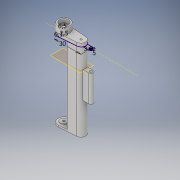
# Autodesk Inventor part: Servo-Arm-Lip
Saved by Autodesk Inventor 2018.3 (Build 223284000, 284)
## iProperties
Created: 2018-02-17
Part Number: Servo-Arm-Lip
Material: Generisch
Document SubType Name: Modeling
Designer: JochenAlt
Density: 1 g/cm^3
Appearance: Vorgabe
Author: JochenAlt
Autodesk Inventor part; units mm, degrees
ref_plane "YZ Plane" through (0, 0, 0) normal (1, 0, 0) x (0, 1, 0)
ref_plane "XZ Plane" through (0, 0, 0) normal (0, 1, 0) x (-1, 0, 0)
sketch "Skizze1" plane through (0, 0, 0) normal (0, 0, 1) x (1, 0, 0)
  line L0 (0, 5.6) -> (0, -5.6) construction
  line L1 (-9.12, 0) -> (26.72, 0) construction
  circle A0 centre (0, 0) radius 2
  circle A1 centre (9.5, 0) radius 1
  circle A2 centre (16, 0) radius 1
  circle A3 centre (19, 0) radius 1
  arc A4 (19.1916, -2.5929) -> (19.1916, 2.5929) centre (19, 0) ccw
  arc A5 (0.2947, 3.9891) -> (0.2947, -3.9891) centre (0, 0) ccw
  line L2 (0.2947, 3.9891) -> (19.1916, 2.5929)
  line L3 (0.2947, -3.9891) -> (19.1916, -2.5929)
  circle A6 centre (12.8, 0) radius 1
  circle A7 centre (0, 0) radius 4
  point P0 (0.5263, 3.9652)
  point P1 (0.6579, -1.8887)
  point P2 (0.6579, 1.8887)
  dimension "d0" = 9.5
  dimension "d1" = 16
  dimension "d2" = 19
  dimension "d3" = 5.2
  dimension "d4" = 2
  dimension "d5" = 4
  dimension "d6" = 8
  dimension "d17" = 12.8
  constraints: 7 centre point, 7 point on circle, 4 coincident, 4 end point, 4 point on line, 4 tangent, 3 equal radius, 3 other
  measures "d0" distance of A1.centre point (0, 0)
  measures "d1" distance of point (0, 0) A2.centre
  measures "d2" distance of A3.centre point (0, 0)
  measures "d3" diameter of A4
  measures "d4" diameter of A3
  measures "d5" diameter of A0
  measures "d6" diameter of A5
  measures "d17" distance of A6.centre point (0, 0)
extrude "Extrusion1" add sketch "Skizze1" along normal blind 1.8
extrude "Extrusion2" add sketch "Skizze1" against normal blind 2.7 contours A5 A7
sketch "Skizze6" plane through (0, 0, 0) normal (0, 0, 1) x (1, 0, 0)
  line L0 (0.2947, 3.9891) -> (19.1916, 2.5929) construction
  arc A0 (19.1916, -2.5929) -> (19.1916, 2.5929) centre (19, 0) ccw construction
  line L1 (19.1916, -2.5929) -> (0.2947, -3.9891) construction
  arc A1 (0.2947, -3.9891) -> (0.2947, 3.9891) centre (0, 0) ccw construction
  circle A2 centre (12.8, 0) radius 1 construction
  circle A3 centre (19, 0) radius 1 construction
  circle A4 centre (16, 0) radius 1 construction
  circle A5 centre (9.5, 0) radius 1 construction
  arc A6 (19.1989, -2.6927) -> (19.1989, 2.6927) centre (19, 0) ccw
  line L2 (19.1989, 2.6927) -> (0.3021, 4.0889)
  line L3 (19.3758, 5.0861) -> (0.4789, 6.4823)
  line L4 (0.4789, -6.4823) -> (19.3758, -5.0861)
  circle A7 centre (9.5, 0) radius 1 construction
  circle A8 centre (19, 0) radius 1
  line L5 (-21.489, 0) -> (83.4343, 0) construction
  arc A9 (0.4789, 6.4823) -> (0.4789, -6.4823) centre (0, 0) ccw
  arc A10 (0.3021, 4.0889) -> (0.3021, -4.0889) centre (0, 0) ccw
  line L6 (0.3021, -4.0889) -> (19.1989, -2.6927)
  circle A11 centre (0, 0) radius 2 construction
  circle A12 centre (0, 0) radius 4.1
  circle A13 centre (0, 0) radius 1.25
  arc A14 (19.3758, -5.0861) -> (19.3758, 5.0861) centre (19, 0) ccw
  line L7 (30, -2.5) -> (23.4452, -2.5)
  arc A15 (30, -2.5) -> (30, 2.5) centre (30, 0) ccw
  line L8 (23.4452, 2.5) -> (30, 2.5)
  circle A16 centre (30, 0) radius 1.5
  dimension "d106" = 2.5
  dimension "d116" = 0.1
  dimension "d198" = 6.5
  dimension "d203" = 5
  dimension "d204" = 30
  dimension "d205" = 3
  constraints: 12 end point, 12 point on circle, 11 centre point, 10 tangent, 8 coincident, 4 concentric, 3 parallel, 1 horizontal, 1 point on line, 1 other
  measures "d106" diameter of A13
  measures "d116" distance between parallel lines of L6 L1
  measures "d198" radius of A9
  measures "d203" diameter of A15
  measures "d204" distance of point (0, 0) A15.centre
  measures "d205" diameter of A16
extrude "Extrusion11" add sketch "Skizze6" along normal blind 2 separate body contours A14 L4 A9 L3
extrude "Extrusion12" add sketch "Skizze6" along normal blind 1.5 from surface at 2 contours L6 A12 L2 A6 | A10 A12 | A14 L4 A9 L3 | A13 bodies 2
extrude "Extrusion16" cut sketch "Skizze6" along normal up to next contours A13 bodies 2
ref_plane "Arbeitsebene8" through (0, 0, -6.75) normal (0, 0, 1) x (1, 0, 0)
sketch "Skizze18" plane through (0, 0, 3.5) normal (0, 0, 1) x (1, 0, 0)
  circle A0 centre (0, 0) radius 5
  circle A1 centre (0, 0) radius 6.5
  circle A2 centre (0, 0) radius 4
  dimension "d183" = 10
  dimension "d192" = 8
  dimension "d197" = 1.5
  constraints: 3 centre point, 3 coincident
  measures "d183" diameter of A0
  measures "d192" diameter of A2
  measures "d197" radial gap between concentric circles of A1 A0
extrude "Extrusion29" add sketch "Skizze18" along normal blind 3 contours A0 | A1 bodies 2
extrude "Extrusion28" add sketch "Skizze18" along normal blind 4 from surface at 3 contours A1 bodies 2
extrude "Extrusion30" add sketch "Skizze6" along normal up to surface (3.5 mm away) contours L6 A12 L2 A6 | A14 L4 A9 L3 bodies 2
sketch "Skizze20" plane through (0, 0, 3.5) normal (0, 0, 1) x (1, 0, 0)
  arc A0 (0.4789, -6.4823) -> (0.4789, 6.4823) centre (0, 0) ccw construction
  line L0 (19.3758, -5.0861) -> (0.4789, -6.4823) construction
  arc A1 (19.3758, -5.0861) -> (19.3758, 5.0861) centre (19, 0) ccw construction
  line L1 (0.4789, 6.4823) -> (19.3758, 5.0861) construction
  circle A2 centre (19, 0) radius 1 construction
  arc A3 (19.3758, -5.0861) -> (19.3758, 5.0861) centre (19, 0) ccw
  line L2 (19.3758, -5.0861) -> (9.403, -5.823)
  line L3 (9.2924, -4.3271) -> (19.2653, -3.5902)
  line L4 (9.403, -5.823) -> (9.2924, -4.3271)
  line L5 (19.3758, 5.0861) -> (16.3839, 5.3072)
  line L6 (0.4789, 6.4823) -> (19.3758, 5.0861) projected
  line L7 (16.3839, 5.3072) -> (16.2734, 3.8113)
  line L8 (16.2734, 3.8113) -> (19.2653, 3.5902)
  arc A4 (19.2653, -3.5902) -> (19.2653, 3.5902) centre (19, 0) ccw
  point P0 (23.4452, -2.5)
  dimension "d221" = 1.5
  dimension "d222" = 3
  dimension "d223" = 10
  constraints: 12 end point, 5 point on circle, 4 tangent, 2 centre point, 2 parallel, 2 perpendicular, 2 point on line, 1 coincident
  measures "d221" distance of L2.end L3.start
  measures "d222" distance of L5.start L5.end
  measures "d223" distance of L2.start L2.end
extrude "Extrusion33" add sketch "Skizze20" against normal blind 88.8 bodies 2
extrude "Extrusion34" add sketch "Skizze6" against normal blind 2 from surface at -85.3 contours L6 A12 L2 A6 | A10 A12 | A14 L4 A9 L3 bodies 2
extrude "Extrusion35" add sketch "Skizze6" along normal blind 0.5 from surface at -85.3 contours A10 A12 bodies 2
ref_plane "Arbeitsebene10" through (0, 0, -22) normal (0, 0, 1) x (1, 0, 0)
extrude "Extrusion36" add sketch "Skizze6" against normal blind 30 from surface at -22 contours L8 A15 L7 A14 bodies 2
